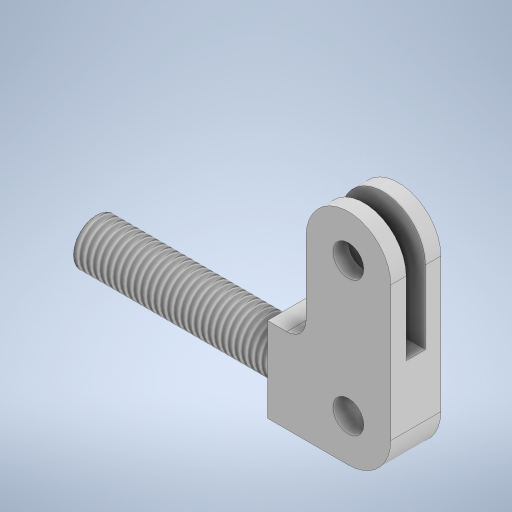
# Autodesk Inventor part: 19_UnionB
Saved by Autodesk Inventor 2024.3 (Build 283343000, 343)
## iProperties
Created: 2024-04-24
Part Number: 19_UnionB
Material: Genérico
Document SubType Name: Modeling
Designer: Cosmic Dinodog
Density: 1 g/cm^3
Appearance: Valor por defecto
Author: Cosmic Dinodog
Autodesk Inventor part; units mm, degrees
ref_plane "YZ Plane" through (0, 0, 0) normal (1, 0, 0) x (0, 1, 0)
ref_plane "XZ Plane" through (0, 0, 0) normal (0, 1, 0) x (-1, 0, 0)
ref_plane "XY Plane" through (0, 0, 0) normal (0, 0, 1) x (1, 0, 0)
sketch "Boceto1" plane through (0, 0, 0) normal (0, 0, 1) x (1, 0, 0)
  circle A0 centre (0, 0) radius 4
  arc A1 (0, -11) -> (11, 0) centre (0, 0) ccw
  line L0 (0, -11) -> (-21, -11)
  line L1 (0, -11) -> (0, 35) construction
  circle A2 centre (0, 35) radius 4
  arc A3 (11, 35) -> (-11, 35) centre (0, 35) ccw
  line L2 (11, 35) -> (11, 0)
  line L3 (-21, -11) -> (-21, 11)
  line L4 (-21, 11) -> (-16, 11)
  line L5 (0, 35) -> (-11, 35) construction
  line L6 (-11, 35) -> (-11, 16)
  arc A4 (-16, 11) -> (-11, 16) centre (-16, 16) ccw
  dimension "d0" = 8
  dimension "d1" = 22
  dimension "d2" = 21
  dimension "d3" = 46
  dimension "d4" = 8
  dimension "d5" = 22
  dimension "d6" = 22
  dimension "d7" = 5
  constraints: 14 end point, 6 point on circle, 6 tangent, 5 centre point, 4 coincident, 3 vertical, 2 horizontal, 1 perpendicular
  measures "d0" diameter of A0
  measures "d1" diameter of A1
  measures "d2" distance of L0.start L0.end
  measures "d3" distance of L0.start L1.end
  measures "d4" diameter of A2
  measures "d5" diameter of A3
  measures "d6" distance of L0.end L3.end
  measures "d7" radius of A4
extrude "Extrusión1" add sketch "Boceto1" against normal blind 13
sketch "Boceto2" plane through (11, 0, 0) normal (1, 0, 0) x (0, 0, -1)
  line L0 (0, 0) -> (4, 0) construction
  line L1 (0, 0) -> (13, 0) construction
  line L2 (0, 35) -> (13, 35) projected
  line L3 (13, 31) -> (0, 31) projected
  line L4 (4, 0) -> (9, 0) construction
  line L5 (13, -11) -> (13, 0) projected
  line L6 (9, 0) -> (13, 0) construction
  line L7 (0, 16) -> (13, 16) construction
  line L8 (4, 16) -> (4, 49.4932)
  line L9 (4, 49.4932) -> (9, 49.4932)
  line L10 (9, 49.4932) -> (9, 16)
  line L11 (4, 16) -> (9, 16)
  line L12 (13, 35) -> (13, 46) projected
  dimension "d10" = 4
  dimension "d11" = 5
  dimension "d12" = 33.4932
  dimension "d13" = 5
  dimension "d14" = 4
  constraints: 14 end point, 4 point on line, 3 perpendicular, 2 collinear
  measures "d10" distance of L0.start L0.end
  measures "d11" distance of L0.end L4.end
  measures "d12" distance of L8.start L8.end
  measures "d13" distance between parallel lines of L8 L10
  measures "d14" distance between parallel lines of L12 L10
extrude "Extrusión2" cut sketch "Boceto2" against normal through all
sketch "Boceto3" plane through (-21, -11, 0) normal (-1, 0, 0) x (0, 0, 1)
  line L0 (-13, 0) -> (-13, 22) projected
  circle A0 centre (-6.5, 11) radius 6
  line L1 (0, 22) -> (-13, 22) projected
  line L2 (-6.5, 22) -> (-6.5, 0) construction
  line L3 (0, 0) -> (-13, 0) projected
  line L4 (0, 11) -> (-13, 11) construction
  line L5 (-13, 11) -> (0, 11)
  dimension "d26" = 12
  constraints: 4 end point, 3 midpoint, 1 centre point, 1 collinear
  measures "d26" diameter of A0
extrude "Extrusión3" add sketch "Boceto3" along normal blind 51
thread "Rosca1" size "M12x1.75" class "6g" standard "ANSI Metric M Profile" full length
chamfer "Chaflán1" distance 0.1 angle 45 1 edges at (-72, 0, -12.5) measured on face at (-72, -0.4786, -4.5581)
